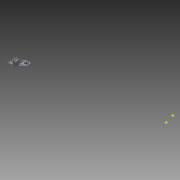
# Autodesk Inventor part: motor-mount
Saved by Autodesk Inventor 2013 (Build 170138000, 138)
## iProperties
Created: 2013-09-28
Part Number: motor-mount
Material: Generic
Document SubType Name: Modeling
Designer: Admin
Density: 1 g/cm^3
Author: Admin
Autodesk Inventor part; units mm, degrees
ref_plane "XZ Plane" through (0, 0, 0) normal (0, 1, 0) x (-1, 0, 0)
ref_plane "XY Plane" through (0, 0, 0) normal (0, 0, 1) x (1, 0, 0)
ref_plane "Work Plane1" through (833.006298, 106.019931, 95.28835) normal (1, 0, 0) x (0, 1, 0)
sketch "Sketch1" plane through (833.006298, 106.019931, 95.28835) normal (1, 0, 0) x (0, 1, 0)
  line L0 (-2.662119, 5.875) -> (-2.662119, 8.25)
  line L1 (-2.662119, 8.25) -> (8.584066, 8.25)
  line L2 (8.584066, 8.25) -> (8.584066, -33.75)
  line L3 (8.584066, -33.75) -> (-2.662119, -33.75)
  line L4 (-2.662119, -33.75) -> (-2.662119, -31.375)
  line L5 (-2.662119, -5.875) -> (-2.662119, -8.25)
  line L6 (-2.662119, -8.25) -> (7.084066, -8.25)
  line L7 (7.084066, -8.25) -> (7.084066, -17.25)
  line L8 (7.084066, -17.25) -> (-2.662119, -17.25)
  line L9 (-2.662119, -17.25) -> (-2.662119, -19.625)
  line L10 (0, 0) -> (3.807, 0)
  line L11 (0, -25.5) -> (3.27539, -25.5)
  arc A0 (-2.662119, -5.875) -> (-2.662119, 5.875) centre (0, 0) ccw
  arc A1 (-2.662119, -31.375) -> (-2.662119, -19.625) centre (0, -25.5) ccw
  point P0 (-106.019931, -95.28835)
  dimension "d0" = 6.45
  dimension "d2" = 6.45
  dimension "d3" = 11.75
  dimension "d4" = 2.375
  dimension "d5" = 1.5
  constraints: 24 end point, 9 collinear, 5 parallel, 4 point on circle, 3 perpendicular, 2 centre point, 2 coincident, 1 vertical, 3 other
  measures "d0" radius of A0
  measures "d2" radius of A1
  measures "d3" distance of L5.start L0.start
  measures "d4" distance from line of L5.start L6
  measures "d5" distance between parallel lines of L2 L7
extrude "Extrusion1" add sketch "Sketch1" against normal blind 20
sketch "Sketch2" plane through (833.006298, 114.603997, 103.53835) normal (0, 1, 0) x (1, 0, 0)
  line L0 (0, 0) -> (0, 42)
  line L1 (0, 42) -> (-20, 42)
  line L2 (-20, 0) -> (-20, 42)
  line L3 (0, 0) -> (-20, 0)
  circle A0 centre (47.06, -29.214085) radius 1.75
  circle A1 centre (24.06, -29.214085) radius 1.75
  circle A2 centre (47.06, -6.214085) radius 1.75
  circle A3 centre (24.06, -6.214085) radius 1.75
  line L4 (20.56, -32.714085) -> (50.56, -32.714085)
  line L5 (50.56, -32.714085) -> (50.56, -2.714085)
  line L6 (-20, 42) -> (-20, 0)
  line L7 (-20, 42) -> (0, 42)
  line L8 (0, 42) -> (50.56, -2.714085)
  line L9 (20.56, -32.714085) -> (-20, 0)
  circle A4 centre (35.56, -17.714085) radius 4
  point P0 (-833.006298, 103.53835)
  dimension "d11" = 3.5
  dimension "d14" = 23
  dimension "d17" = 23
  dimension "d20" = 11.5
  dimension "d21" = 11.5
  dimension "d22" = 30
  dimension "d23" = 30
  dimension "d24" = 15
  dimension "d25" = 15
  dimension "d26" = 8
  constraints: 12 end point, 5 centre point, 2 collinear, 1 coincident, 1 horizontal, 1 parallel, 1 perpendicular, 1 vertical, 6 other
  measures "d11" diameter of A0
  measures "d14" distance of A0.centre A1.centre
  measures "d17" distance of A0.centre A2.centre
  measures "d20" horizontal distance of point (35.56, -17.714) A0.centre
  measures "d21" horizontal distance of point (35.56, -17.714) A0.centre
  measures "d22" distance of L4.end L5.end
  measures "d23" distance of L4.start L4.end
  measures "d24" distance from line of point (35.56, -17.714) L5
  measures "d25" distance from line of point (35.56, -17.714) L4
  measures "d26" diameter of A4
extrude "Extrusion2" add sketch "Sketch2" against normal up to surface (1.5 mm away) contours L0 L8 L5 L4 L9 L3
ref_plane "Work Plane2" through (848.006298, 50.269931, 288.96335) normal (1, 0, 0) x (0, 0.9453708, -0.3259971)
ref_plane "Work Plane3" through (833.006298, 106.019931, 95.28835) normal (0, -1, 0) x (-1, 0, 0)
ref_plane "Work Plane6" through (833.006298, 86.019931, 69.78835) normal (0, -0.986957, -0.1609842) x (1, 0, 0)
ref_plane "Work Plane7" through (833.006298, 106.019931, 95.28835) normal (0, 0.1609842, -0.986957) x (-1, 0, 0)
sketch "Sketch4" plane through (833.006298, 106.019931, 95.28835) normal (0, 0.1609842, -0.986957) x (-1, 0, 0)
  line L0 (-9.125, -26.717558) -> (-6.75, -26.717558)
  line L1 (-6.75, -26.717558) -> (-6.75, 8.282442)
  line L2 (-6.75, 8.282442) -> (-23.25, 8.282442)
  line L3 (-23.25, 8.282442) -> (-23.25, -26.717558)
  line L4 (-23.25, -26.717558) -> (-20.875, -26.717558)
  line L5 (-15, -23.844237) -> (-15, 8.282442)
  arc A0 (-9.125, -26.717558) -> (-20.875, -26.717558) centre (-15, -23.844237) ccw
  point P0 (833.006298, -119.97703)
  dimension "d31" = 11.75
  dimension "d33" = 2.375
  dimension "d34" = 6.54
  dimension "d35" = 35
  constraints: 12 end point, 2 collinear, 2 parallel, 2 perpendicular, 2 point on circle, 1 centre point, 1 coincident, 1 horizontal, 1 midpoint, 1 other
  measures "d31" distance of L0.start L4.end
  measures "d33" distance of L3.end L4.end
  measures "d34" radius of A0
  measures "d35" distance of L0.end L1.end
extrude "Extrusion3" add sketch "Sketch4" along normal up to surface surface through (833.006298, 114.603997, 103.53835) normal (0, 1, 0)
sketch "Sketch6" plane through (856.256298, 114.603997, 82.100108) normal (0, 1, 0) x (1, 0, 0)
  line L0 (0, 0) -> (-16.5, 14.592215)
  line L1 (0, 205.402536) -> (0, 0)
  line L2 (-2.375, 205.402536) -> (0, 205.402536)
  ellipse E0 centre (-8.25, 187.554069) end of major axis (-8.25, 146.928964) minor radius 6.54 (-2.375, 205.402536) -> (-14.125, 205.402536) ccw
  line L3 (-16.5, 205.402536) -> (-14.125, 205.402536)
  line L4 (-16.5, 14.592215) -> (-16.5, 205.402536)
  point P0 (-856.256298, 82.100108)
  constraints: 1 other
extrude "Extrusion5" cut sketch "Sketch6" against normal through all
sketch "Sketch7" plane through (853.566298, 114.603997, 136.252436) normal (0, 1, 0) x (1, 0, 0)
  circle A0 centre (26.5, 3.5) radius 1.75
  circle A1 centre (3.5, 3.5) radius 1.75
  circle A2 centre (26.5, 26.5) radius 1.75
  circle A3 centre (3.5, 26.5) radius 1.75
  circle A4 centre (15, 15) radius 4
  line L0 (-20.56, 74.714085) -> (-40.56, 74.714085)
  line L1 (-40.56, 32.714085) -> (-40.56, 74.714085)
  line L2 (-40.56, 32.714085) -> (0, 0)
  line L3 (0, 0) -> (30, 0)
  line L4 (30, 0) -> (30, 30)
  line L5 (30, 30) -> (-20.56, 74.714085)
  circle A5 centre (15, 15) radius 11.25
  point P0 (-853.566298, 136.252436)
  dimension "d56" = 22.5
  constraints: 1 centre point, 1 coincident
  measures "d56" diameter of A5
extrude "Extrusion6" add sketch "Sketch7" along normal blind 2.5 contours L5 L4 L3 L2 L1 L0
sketch "Sketch8" plane through (813.006298, 113.103997, 87.03835) normal (0, -1, 0) x (1, 0, 0)
  line L0 (20, 0) -> (20, 16.5)
  line L1 (20, -25.5) -> (20, -9)
  line L2 (26.75, -19.530457) -> (20, -25.5)
  line L3 (20, 16.5) -> (21, 16.5)
  line L4 (20, -9) -> (21, -9)
  line L5 (20, 0) -> (21, 0)
  line L6 (21, 16.5) -> (21, 0)
  line L7 (21, -9) -> (21, -24.615623)
  point P0 (-813.006298, -87.03835)
  dimension "d59" = 1
  constraints: 10 end point, 5 perpendicular, 1 parallel, 1 point on line
  measures "d59" distance of L0.end L3.end
extrude "Extrusion7" add sketch "Sketch8" along normal up to surface (4.873092 mm away)
fillet "Fillet1" radius 2 12 edges at (856.2563, 113.104, 89.272) (834.0063, 113.104, 70.2305) (833.0063, 108.2309, 62.6337) (833.0063, 108.2309, 76.943) (823.5063, 113.104, 87.0384) (833.0063, 108.2309, 88.1337) (823.5063, 113.104, 78.0384) (839.7563, 113.104, 81.9759) (823.5063, 113.104, 103.5384) (834.0063, 113.104, 95.2884) (848.0063, 113.104, 96.4438) (833.0063, 108.2309, 102.443)
sketch "Sketch9" plane through (868.566298, 114.603997, 121.252436) normal (0, 1, 0) x (1, 0, 0)
  circle A0 centre (0, 0) radius 11.25 projected
  circle A1 centre (0, 0) radius 4 projected
  point P0 (-868.566298, 121.252436)
extrude "Extrusion8" cut sketch "Sketch9" against normal through all
sketch "Sketch10" plane through (853.566298, 113.103997, 136.252436) normal (0, -1, 0) x (1, 0, 0)
  line L0 (4.69, -38.108384) -> (-15.81, -38.108384)
  line L1 (4.69, -52.383574) -> (4.69, -38.108384)
  line L2 (30, -30) -> (4.69, -52.383574)
  line L3 (-38.080334, -30.714085) -> (0, 0)
  line L4 (-17.56, -30.714085) -> (-38.080334, -30.714085)
  line L5 (-17.56, -51.214085) -> (-17.56, -30.714085)
  line L6 (0, 0) -> (0, -30)
  line L7 (0, -30) -> (30, -30)
  line L8 (-15.81, -38.108384) -> (-17.56, -38.108384)
  line L9 (-27.377388, -25.935714) -> (-4.627804, -7.586802)
  line L10 (9.352474, -44.255307) -> (20.101537, -34.749085)
  line L11 (-26.749584, -27.714085) -> (-15.56, -27.714085)
  line L12 (-14.56, -28.714085) -> (-14.56, -34.108384)
  line L13 (-13.56, -35.108384) -> (-4, -35.108384)
  line L14 (-3, -34.108384) -> (-3, -8.365174)
  line L15 (3, -34) -> (3, -34.108384)
  line L16 (4, -35.108384) -> (6.69, -35.108384)
  line L17 (7.69, -36.108384) -> (7.69, -43.506221)
  line L18 (4, -33) -> (19.439064, -33)
  arc A0 (-27.377388, -25.935714) -> (-26.749584, -27.714085) centre (-26.749584, -26.714085) ccw
  arc A1 (-14.56, -28.714085) -> (-15.56, -27.714085) centre (-15.56, -28.714085) ccw
  arc A2 (-14.56, -34.108384) -> (-13.56, -35.108384) centre (-13.56, -34.108384) ccw
  arc A3 (-4, -35.108384) -> (-3, -34.108384) centre (-4, -34.108384) ccw
  arc A4 (-3, -8.365174) -> (-4.627804, -7.586802) centre (-4, -8.365174) ccw
  arc A5 (4, -33) -> (3, -34) centre (4, -34) ccw
  arc A6 (3, -34.108384) -> (4, -35.108384) centre (4, -34.108384) ccw
  arc A7 (7.69, -36.108384) -> (6.69, -35.108384) centre (6.69, -36.108384) ccw
  arc A8 (7.69, -43.506221) -> (9.352474, -44.255307) centre (8.69, -43.506221) ccw
  arc A9 (20.101537, -34.749085) -> (19.439064, -33) centre (19.439064, -34) ccw
  point P0 (-853.566298, -136.252436)
  dimension "d65" = 1
  dimension "d66" = 3
  dimension "d67" = 3
  dimension "d68" = 3
  dimension "d69" = 3
  dimension "d70" = 3
  dimension "d71" = 3
  dimension "d72" = 3
  dimension "d73" = 3
  dimension "d74" = 3
  dimension "d77" = 3
  constraints: 26 end point, 20 point on circle, 20 tangent, 10 centre point, 9 equal radius, 7 parallel, 6 perpendicular, 1 point on line
  measures "d65" radius of A0
  measures "d66" distance between parallel lines of L3 L9
  measures "d67" distance between parallel lines of L2 L10
  measures "d68" distance between parallel lines of L18 L7
  measures "d69" distance between parallel lines of L6 L14
  measures "d70" distance between parallel lines of L0 L13
  measures "d71" distance between parallel lines of L5 L12
  measures "d72" distance between parallel lines of L4 L11
  measures "d73" distance between parallel lines of L1 L17
  measures "d74" distance between parallel lines of L6 L15
  measures "d77" distance between parallel lines of L16 L0
extrude "Extrusion9" cut sketch "Sketch10" against normal through all contours L9 A4 L14 A3 L13 A2 L12 A1 L11 A0 | A8 L17 A7 L16 A6 L15 A5 L18 A9 L10
move or copy body "Move Body1" bodies to move or copy 1 copy no rotation origin (0, 0, 0) rotation axis (1, 0, 0) rotation angle -90 translate (0, 41.819462, 164.896163)
move or copy body "Move Body2" bodies to move or copy 1 copy no translate (-813.006298, -103.357812, -47.792166)
move or copy body "Move Body3" bodies to move or copy 1 copy no translate (10, 0, 0)
move or copy body "Move Body4" bodies to move or copy 1 copy no translate (-36.75, 0, 0)
ref_plane "Work Plane4" through (833.006298, 86.019931, 95.28835) normal (0, -1, 0) x (-1, 0, 0)
ref_plane "Work Plane5" through (833.006298, 106.019931, 69.78835) normal (0, 0, 1) x (-1, 0, 0)
equation "\"d2\" = d0"
equation "\"d20\" = 0.5 * d14"
equation "\"d21\" = 0.5 * d17"
equation "\"d23\" = d22"
equation "\"d24\" = 0.5 * d22"
equation "\"d25\" = 0.5 * d23"
equation "\"d67\" = d66"
equation "\"d68\" = d66"
equation "\"d69\" = d66"
equation "\"d70\" = d66"
equation "\"d71\" = d66"
equation "\"d72\" = d66"
equation "\"d73\" = d72"
equation "\"d74\" = d73"
equation "\"d77\" = d73"
body "Solid1"
